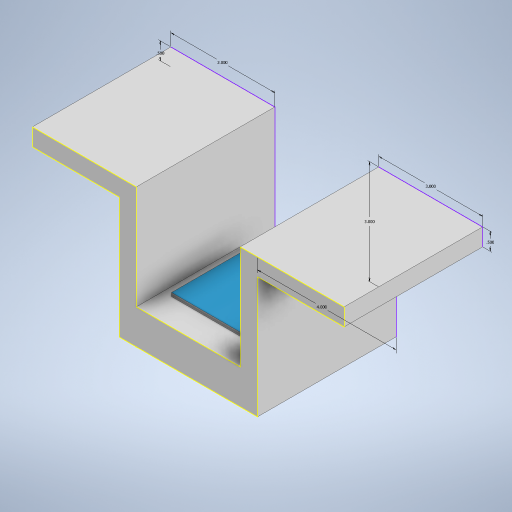
# Autodesk Inventor part: Chassis
Saved by Autodesk Inventor 2023 (Build 270158000, 158)
## iProperties
Created: 2023-09-27
Part Number: Chassis
Material: Generic
Document SubType Name: Modeling
Designer: Turnt
Density: 1 g/cm^3
Appearance: Default
Author: Turnt
Autodesk Inventor part; units mm, degrees
ref_plane "YZ Plane" through (0, 0, 0) normal (1, 0, 0) x (0, 1, 0)
ref_plane "XZ Plane" through (0, 0, 0) normal (0, 1, 0) x (-1, 0, 0)
ref_plane "XY Plane" through (0, 0, 0) normal (0, 0, 1) x (1, 0, 0)
sketch "Sketch1" plane through (0, 0, 0) normal (0, 0, 1) x (1, 0, 0)
  line L0 (0, 0) -> (76.2, 0)
  line L1 (76.2, 25.4) -> (0, 25.4)
  line L2 (76.2, 25.4) -> (76.2, 101.6)
  line L3 (76.2, 101.6) -> (152.4, 101.6)
  line L4 (152.4, 101.6) -> (152.4, 88.9)
  line L5 (88.9, 88.9) -> (88.9, 25.4)
  line L6 (88.9, 88.9) -> (152.4, 88.9)
  line L7 (88.9, 25.4) -> (88.9, 0)
  line L8 (88.9, 0) -> (76.2, 0)
  line L9 (0, 0) -> (-12.7, 0)
  line L10 (-12.7, 0) -> (-12.7, 88.9)
  line L11 (0, 101.6) -> (0, 25.4)
  line L12 (-76.2, 101.6) -> (-76.2, 88.9)
  line L13 (-76.2, 88.9) -> (-12.7, 88.9)
  line L14 (-76.2, 101.6) -> (0, 101.6)
  dimension "d4" = 76.2
  dimension "d5" = 76.2
  dimension "d6" = 12.7
  dimension "d11" = 76.2
  dimension "d12" = 12.7
  dimension "d13" = 101.6
  constraints: 30 end point, 4 perpendicular, 3 horizontal, 2 vertical, 1 parallel, 1 point on line
  measures "d4" distance of L1.start L2.end
  measures "d5" distance of L2.end L3.end
  measures "d6" distance of L3.end L4.end
  measures "d11" distance of L12.start L11.start
  measures "d12" distance of L12.start L12.end
  measures "d13" distance of L7.end L9.end
extrude "Extrusion1" add sketch "Sketch1" along normal blind 101.6
sketch "Sketch2" plane through (0, 25.4, 0) normal (0, 1, 0) x (1, 0, 0)
  line L0 (76.2, 0) -> (0, 0) projected
  line L1 (0, 0) -> (0, -101.6) projected
  line L2 (76.2, -101.6) -> (0, -101.6) projected
  line L3 (76.2, 0) -> (76.2, -101.6) projected
  line L4 (69.85, -18.6469) -> (6.35, -18.6469)
  line L5 (6.35, -18.6469) -> (6.35, -82.1469)
  line L6 (6.35, -82.1469) -> (69.85, -82.1469)
  line L7 (69.85, -82.1469) -> (69.85, -18.6469)
  line L8 (69.85, -18.6469) -> (6.35, -82.1469) construction
  line L9 (6.35, -18.6469) -> (69.85, -82.1469) construction
  point P0 (38.1, -50.3969)
  dimension "d16" = 63.5
  dimension "d17" = 63.5
  constraints: 12 end point, 2 midpoint, 2 parallel, 1 horizontal, 1 perpendicular
  measures "d16" distance of L6.end L5.end
  measures "d17" distance of L5.end L4.end
extrude "Extrusion2" add sketch "Sketch2" along normal blind 2.54 contours L7 L6 L5 L4
sketch "Sketch3" plane through (0, 0, 101.6) normal (0, 0, 1) x (1, 0, 0)
  line L0 (-12.7, 0) -> (88.9, 0) projected
  line L1 (88.9, 0) -> (88.9, 88.9) projected
  line L2 (88.9, 88.9) -> (152.4, 88.9) projected
  line L3 (152.4, 88.9) -> (152.4, 101.6) projected
  line L4 (152.4, 101.6) -> (76.2, 101.6) projected
  line L5 (76.2, 101.6) -> (76.2, 25.4) projected
  line L6 (76.2, 25.4) -> (0, 25.4) projected
  line L7 (0, 25.4) -> (0, 101.6) projected
  line L8 (0, 101.6) -> (-76.2, 101.6) projected
  line L9 (-76.2, 101.6) -> (-76.2, 88.9) projected
  line L10 (-76.2, 88.9) -> (-12.7, 88.9) projected
  line L11 (-12.7, 88.9) -> (-12.7, 0) projected
  point P0 (0, 0)
body "Solid1"
